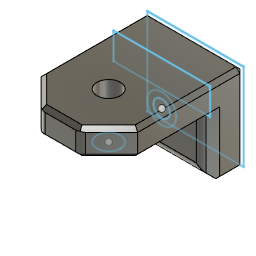
Mount (Autodesk Fusion 360 design; units mm, degrees)
Autodesk Fusion 360 part; units mm, degrees
sketch "sketch 738" plane through (0, 380, 0) normal (0, -1, 0) x (1, 0, 0)
  line L0 (-185.0624, -39) -> (-185.0624, -21)
  line L1 (-185.0624, -21) -> (-205.0624, -21)
  line L2 (-185.0624, -21) -> (-205.0624, -21)
  line L3 (-205.0624, -21) -> (-205.0624, -39)
  line L4 (-205.0624, -39) -> (-185.0624, -39)
extrude "Extrude1" add sketch "sketch 738" along normal blind 7
sketch "sketch 788" plane through (0, 373, 0) normal (0, -1, 0) x (1, 0, 0)
  line L0 (-185.0624, -26.5) -> (-205.0624, -26.5)
  line L1 (-185.0624, -21) -> (-185.0624, -26.5)
  line L2 (-185.0624, -21) -> (-185.0624, -26.5)
  line L3 (-205.0624, -21) -> (-185.0624, -21)
  line L4 (-205.0624, -21) -> (-185.0624, -21)
  line L5 (-205.0624, -26.5) -> (-205.0624, -21)
  line L6 (-205.0624, -26.5) -> (-205.0624, -21)
extrude "Extrude4" add sketch "sketch 788" along normal blind 21
sketch "sketch 773" plane through (0, 373, 0) normal (0, -1, 0) x (1, 0, 0)
  circle A0 centre (-195.0624, -30) radius 1.7
  circle A1 centre (-195.0624, -30) radius 3
extrude "Extrude3" cut sketch "sketch 773" against normal blind 3
sketch "sketch 761" plane through (0, 373, 0) normal (0, -1, 0) x (1, 0, 0)
  circle A0 centre (-195.0624, -30) radius 1.7
extrude "Extrude2" cut sketch "sketch 761" against normal blind 7
sketch "sketch 812" plane through (0, 0, -30.5) normal (0, 0, -1) x (1, 0, 0)
  circle A0 centre (-195.0624, -362) radius 2.425
extrude "Extrude5" cut sketch "sketch 812" against normal blind 10
fillet "Fillet1" [suppressed]
chamfer "Chamfer2" distance 2 angle 45 3 edges at (-205.0624, 373, -32.75) (-195.0624, 373, -39) (-185.0624, 373, -32.75)
fillet "Fillet2" radius 2 3 edges at (-203.0624, 373, -31.75) (-195.0624, 373, -37) (-187.0624, 373, -31.75)
chamfer "Chamfer4" distance 6 angle 45 2 edges at (-185.0624, 352, -23.75) (-205.0624, 352, -23.75)
chamfer "Chamfer5" distance 0.8 angle 45 12 edges at (-185.0624, 369, -21) (-185.0624, 366.5, -26.5) (-188.0624, 355, -21) (-188.0624, 355, -26.5) (-195.0624, 352, -26.5) (-195.0624, 352, -21) (-202.0624, 355, -21) (-202.0624, 355, -26.5) (-205.0624, 369, -21) (-205.0624, 366.5, -26.5) (-185.0624, 377.5, -39) (-205.0624, 377.5, -39) 1 faces at (-202.2958, 380, -30)
fillet "Fillet3" radius 2 2 edges at (-191.0624, 352, -23.75) (-199.0624, 352, -23.75)
named bodies: "Tube mount"
